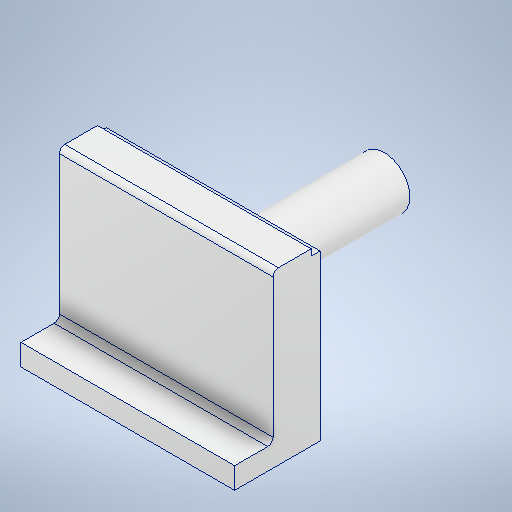
# Autodesk Inventor part: Molde
Saved by Autodesk Inventor 2025.1 (Build 291241000, 241)
## iProperties
Created: 2025-01-29
Part Number: Molde
Material: Aluminum 6061
Document SubType Name: Modeling
Designer: yovan
Mass: 52137.2 g
Surface Area: 6362.53 cm^2
Volume: 19310.1 cm^3
Density: 2.7 g/cm^3
Appearance: Aluminum - Flat
Author: yovan
Autodesk Inventor part; units mm, degrees
ref_plane "YZ Plane" through (0, 0, 0) normal (1, 0, 0) x (0, 1, 0)
ref_plane "XZ Plane" through (0, 0, 0) normal (0, 1, 0) x (-1, 0, 0)
ref_plane "XY Plane" through (0, 0, 0) normal (0, 0, 1) x (1, 0, 0)
sketch "Sketch1" plane through (0, 0, 0) normal (1, 0, 0) x (0, 1, 0)
  line L0 (400, 120) -> (0, 120)
  line L1 (0, 40) -> (0, 62.8571)
  line L2 (400, 120) -> (0, 120)
  line L3 (0, 120) -> (0, 30)
  line L4 (0, 30) -> (400, 30)
  line L5 (400, 30) -> (400, 120)
  dimension "d54" = 400
  dimension "d55" = 90
  constraints: 12 end point, 2 parallel, 1 horizontal, 1 perpendicular
  measures "d54" distance of L0.start L0.end
  measures "d55" distance of L4.end L0.start
extrude "Extrusion1" add sketch "Sketch1" along normal blind 500
sketch "Sketch2" plane through (500, 0, 0) normal (1, 0, 0) x (0, 0, -1)
  line L0 (-30, 400) -> (80, 400)
  line L1 (80, 400) -> (80, 350)
  line L2 (80, 350) -> (-30, 350)
  line L3 (-30, 350) -> (-30, 400)
  arc A0 (-42.5, 0) -> (-30, 12.5) centre (-42.5, 12.5) ccw
  line L4 (-120, 0) -> (-30, 0) projected
  line L5 (-30, 0) -> (-64.3382, 0)
  line L6 (-30, 12.5) -> (-30, 0)
  line L7 (-120, 400) -> (-120, 0) projected
  line L8 (-120, 0) -> (-70, 0)
  line L9 (-70, 0) -> (-70, 50)
  line L10 (-70, 50) -> (-120, 50)
  line L11 (-120, 50) -> (-120, 0)
  point P0 (-70, 0)
  dimension "d11" = 110
  dimension "d12" = 50
  dimension "d33" = 12.5
  dimension "d38" = 50
  dimension "d39" = 50
  constraints: 20 end point, 4 parallel, 3 horizontal, 2 perpendicular, 2 point on circle, 1 centre point
  measures "d11" distance of L1.end L2.end
  measures "d12" distance of L0.end L1.end
  measures "d33" radius of A0
  measures "d38" distance of L10.end L9.end
  measures "d39" distance of L9.end L8.end
extrude "Extrusion11" cut sketch "Sketch2" against normal blind 500 contours A0 L6 L4
extrude "Extrusion12" add sketch "Sketch2" against normal blind 500 contours L0 L1 L2 L3
sketch "Sketch8" plane through (0, 0, 120) normal (0, 0, 1) x (1, 0, 0)
  line L0 (0, 0) -> (500, 0) projected
  line L1 (0, 400) -> (500, 400) projected
  line L2 (0, 0) -> (500, 0)
  line L3 (500, 0) -> (500, 400)
  line L4 (500, 400) -> (0, 400)
  line L5 (0, 400) -> (0, 0)
  line L6 (264, 195) -> (236, 195)
  line L7 (235, 194) -> (235, 166)
  line L8 (236, 165) -> (264, 165)
  line L9 (265, 166) -> (265, 194)
  arc A0 (236, 195) -> (235, 194) centre (236, 194) ccw
  arc A1 (265, 194) -> (264, 195) centre (264, 194) ccw
  arc A2 (264, 165) -> (265, 166) centre (264, 166) ccw
  arc A3 (235, 166) -> (236, 165) centre (236, 166) ccw
  point P0 (265, 195)
  point P1 (235, 165)
  point P2 (235, 195)
  point P3 (265, 165)
  dimension "d77" = 30
  dimension "d78" = 30
  dimension "d83" = 1
  constraints: 16 end point, 8 point on circle, 8 point on line, 8 tangent, 4 centre point, 4 parallel, 3 equal radius, 2 horizontal, 2 perpendicular
  measures "d77" distance of point (265, 165) point (235, 165)
  measures "d78" distance of point (235, 165) point (235, 195)
  measures "d83" radius of A0
extrude "Extrusion17" cut sketch "Sketch8" against normal blind 90 contours A1 L9 A2 L8 A3 L7 A0 L6
sketch "Sketch10" plane through (500, 12.5, 30) normal (0, 0, -1) x (-1, 0, 0)
  line L0 (236, 152.5) -> (264, 152.5)
  line L1 (265, 153.5) -> (265, 201.5)
  line L2 (264, 202.5) -> (236, 202.5)
  line L3 (235, 201.5) -> (235, 153.5)
  arc A0 (236, 202.5) -> (235, 201.5) centre (236, 201.5) ccw
  arc A1 (265, 201.5) -> (264, 202.5) centre (264, 201.5) ccw
  arc A2 (264, 152.5) -> (265, 153.5) centre (264, 153.5) ccw
  arc A3 (235, 153.5) -> (236, 152.5) centre (236, 153.5) ccw
  point P0 (500, -12.5)
  point P1 (265, 202.5)
  point P2 (265, 152.5)
  point P3 (235, 202.5)
  dimension "d84" = 30
  dimension "d85" = 50
  dimension "d86" = 1
  constraints: 8 end point, 8 point on circle, 8 tangent, 6 point on line, 4 centre point, 3 equal radius, 2 parallel, 1 horizontal, 1 perpendicular
  measures "d84" distance of point (235, 202.5) point (265, 202.5)
  measures "d85" distance of point (265, 202.5) point (265, 152.5)
  measures "d86" radius of A0
extrude "Extrusion18" cut sketch "Sketch10" against normal blind 15
fillet "Face Fillet1" radius 12.5 1 edges at (250, 350, 30)
sketch "Sketch11" plane through (0, 350, -80) normal (0, -1, 0) x (1, 0, 0)
  line L0 (500, 0) -> (0, 0) projected
  line L1 (500, 0) -> (0, 0)
  line L2 (0, 0) -> (0, 20)
  line L3 (0, 20) -> (500, 20)
  line L4 (500, 20) -> (500, 0)
  dimension "d92" = 500
  dimension "d93" = 20
  constraints: 8 end point, 2 parallel, 1 horizontal, 1 perpendicular
  measures "d92" distance of L2.end L3.end
  measures "d93" distance of L1.end L2.end
extrude "Extrusion19" add sketch "Sketch11" along normal blind 15
fillet "Face Fillet2" radius 1 1 edges at (250, 350, -60)
fillet "Face Fillet3" radius 1 1 edges at (250, 335, -60)
sketch "Sketch12" plane through (0, 400, 120) normal (0, 1, 0) x (1, 0, 0)
  line L0 (0, 0) -> (500, 0) projected
  line L1 (500, 200) -> (0, 200) projected
  line L2 (0, 0) -> (500, 0)
  line L3 (500, 0) -> (500, 200)
  line L4 (500, 200) -> (0, 200)
  line L5 (0, 200) -> (0, 0)
  point P0 (0, 120)
  constraints: 8 end point, 2 parallel, 1 horizontal, 1 perpendicular
extrude "Extrusion20" add sketch "Sketch12" against normal blind 450 separate body
combine bodies "Combine1" operation type subtract main body 2 bodies to subtract 1
sketch "Sketch13" plane through (265, 166, 30) normal (1, 0, 0) x (0, 0, -1)
  line L0 (0, 171.5) -> (0, -153.5) projected
  line L1 (0, 82.5169) -> (-114.772, 82.5169)
  line L2 (-114.772, 82.5169) -> (-114.772, -52.2022)
  line L3 (-114.772, -52.2022) -> (0, -52.2022)
  line L4 (0, -52.2022) -> (0, 82.5169)
  point P0 (30, -166)
  point P1 (0, -52.2022)
  constraints: 8 end point, 2 parallel, 1 horizontal, 1 perpendicular, 1 point on line
extrude "Extrusion21" cut sketch "Sketch13" against normal blind 150 bodies 2
sketch "Sketch14" plane through (500, -50, -80) normal (0, 0, -1) x (-1, 0, 0)
  circle A0 centre (250, 200) radius 60
  dimension "d104" = 120
  constraints: 1 centre point
  measures "d104" diameter of A0
extrude "Extrusion22" add sketch "Sketch14" along normal blind 400 bodies 2
body "Solid2"
